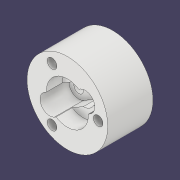
# Autodesk Inventor part: AA050
Saved by Autodesk Inventor 2017 SP1 (Build 210196100, 196)
## iProperties
Created: 2018-02-16
Part Number: AA050
Material: ABS Plastic
Document SubType Name: Modeling
Designer: Zach
Density: 1.06 g/cm^3
Appearance: CR White
Author: Zach
Autodesk Inventor part; units mm, degrees
ref_plane "YZ Plane" through (0, 0, 0) normal (1, 0, 0) x (0, 1, 0)
ref_plane "XZ Plane" through (0, 0, 0) normal (0, 1, 0) x (-1, 0, 0)
ref_plane "XY Plane" through (0, 0, 0) normal (0, 0, 1) x (1, 0, 0)
sketch "Sketch1" plane through (0, 0, 0) normal (0, 0, 1) x (1, 0, 0)
  circle A0 centre (0, 0) radius 12.5
  circle A1 centre (0, 0) radius 3.5
  circle A2 centre (9.525, 0) radius 1.5
  circle A3 centre (-4.7625, 8.2489) radius 1.5
  circle A4 centre (-4.7625, -8.2489) radius 1.5
  circle A5 centre (5.4993, 3.175) radius 1.5
  line L0 (0, 0) -> (5.4993, 3.175) construction
  line L1 (0, 0) -> (17.6195, 0) construction
  circle A6 centre (-5.4993, -3.175) radius 1.5
  dimension "d0" = 25
  dimension "d1" = 7
  dimension "d2" = 3
  dimension "d3" = 9.525
  dimension "d6" = 360
  dimension "d8" = 3
  dimension "d10" = 6.35
  dimension "d11" = 30
  dimension "d14" = 360
  constraints: 7 centre point, 4 end point, 2 coincident, 1 horizontal, 1 horizontal alignment, 12 other
  measures "d0" diameter of A0
  measures "d1" diameter of A1
  measures "d2" diameter of A2
  measures "d3" distance of A2.centre point (0, 0)
  measures "d8" diameter of A5
  measures "d10" distance of L0.start L0.end
  measures "d11" angle of L0 L1
extrude "Extrusion1" add sketch "Sketch1" along normal blind 14
sketch "Sketch5" plane through (0, 0, 14) normal (0, 0, 1) x (1, 0, 0)
  circle A0 centre (5.4993, 3.175) radius 3
  circle A1 centre (-5.4993, -3.175) radius 3
  circle A2 centre (5.4993, 3.175) radius 1.5 projected
  circle A3 centre (-5.4993, -3.175) radius 1.5 projected
  dimension "d23" = 6
  dimension "d24" = 6
  constraints: 2 centre point, 2 coincident
  measures "d23" diameter of A0
  measures "d24" diameter of A1
extrude "Extrusion3" cut sketch "Sketch5" against normal blind 9 contours A0 | A1 | A2 | A3
sketch "Sketch2" plane through (0, 0, 14) normal (0, 0, 1) x (1, 0, 0)
  circle A0 centre (0, 0) radius 3.5 construction
  line L0 (0, 8.6603) -> (7.5, 4.3301)
  line L1 (7.5, 4.3301) -> (7.5, -4.3301)
  line L2 (7.5, -4.3301) -> (0, -8.6603)
  line L3 (0, -8.6603) -> (-7.5, -4.3301)
  line L4 (-7.5, -4.3301) -> (-7.5, 4.3301)
  line L5 (-7.5, 4.3301) -> (0, 8.6603)
  circle A1 centre (9.525, 0) radius 1.5 construction
  line L6 (0, 0) -> (9.525, 0) construction
  point P0 (7.5, 0)
  dimension "d18" = 15
  constraints: 14 end point, 1 coincident, 1 horizontal, 1 midpoint, 1 point on line, 13 other
  measures "d18" distance between parallel lines of L2 L5
extrude "Extrusion2" [suppressed]
sketch "Sketch6" plane through (0, 0, 14) normal (0, 0, 1) x (1, 0, 0)
  circle A0 centre (0, 0) radius 6.5
  dimension "d27" = 13
  constraints: 1 centre point, 1 coincident
  measures "d27" diameter of A0
extrude "Extrusion4" cut sketch "Sketch6" against normal blind 5
sketch "Sketch7" plane through (0, 0, 5) normal (0, 0, 1) x (1, 0, 0)
  arc A0 (-3.3173, -1.1161) -> (-2.6252, -2.3148) centre (0, 0) ccw projected
  arc A1 (-3.3173, -1.1161) -> (-2.6252, -2.3148) centre (-5.4993, -3.175) ccw projected
  circle A2 centre (-5.4993, -3.175) radius 1.5 projected
  circle A3 centre (5.4993, 3.175) radius 1.5 projected
  arc A4 (3.3173, 1.1161) -> (2.6252, 2.3148) centre (0, 0) ccw projected
  arc A5 (3.3173, 1.1161) -> (2.6252, 2.3148) centre (5.4993, 3.175) ccw projected
  circle A6 centre (5.4993, 3.175) radius 1.5 projected
  line L0 (-6.9993, -0.5769) -> (3.9993, 5.7731)
  line L1 (-3.9993, -5.7731) -> (6.9993, 0.5769)
  arc A7 (6.9993, 0.5769) -> (3.9993, 5.7731) centre (5.4993, 3.175) ccw
  arc A8 (-6.9993, -0.5769) -> (-3.9993, -5.7731) centre (-5.4993, -3.175) ccw
  constraints: 8 point on circle, 6 tangent, 4 end point, 2 centre point, 1 concentric
extrude "Extrusion5" cut sketch "Sketch7" along normal through all contours A1 L0 A5 A4 L1 A0 | A0 A1 | A5 A4 | A2 | A3
body "Solid1"
